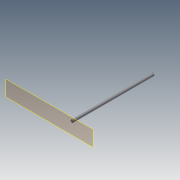
# Autodesk Inventor part: Shaft
Saved by Autodesk Inventor 2014 SP1 (Build 180222100, 222)
## iProperties
Created: 2014-03-25
Part Number: Shaft
Material: Generic
Document SubType Name: Modeling
Designer: tom
Density: 1 g/cm^3
Appearance: Default
Author: tom
Autodesk Inventor part; units mm, degrees
ref_plane "YZ Plane" through (0, 0, 0) normal (1, 0, 0) x (0, 1, 0)
ref_plane "XZ Plane" through (0, 0, 0) normal (0, 1, 0) x (-1, 0, 0)
ref_plane "XY Plane" through (0, 0, 0) normal (0, 0, 1) x (1, 0, 0)
ref_plane "Work Plane1" through (-41.7705, -13.51, -28.1343) normal (0, 0, 1) x (1, 0, 0)
sketch "Sketch1" plane through (-41.7705, -13.51, -28.1343) normal (0, 0, 1) x (1, 0, 0)
  circle A0 centre (70.5, 13) radius 1.125 projected
  circle A1 centre (70.5, 13) radius 1.5
  point P0 (41.7705, 13.51)
  dimension "d0" = 3
  constraints: 1 centre point, 1 coincident
  measures "d0" diameter of A1
extrude "Extrusion1" add sketch "Sketch1" against normal blind 91.5 contours A0 | A1
body "Solid1"
